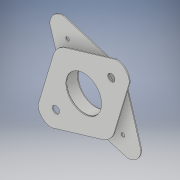
# Autodesk Inventor part: Dampner
Saved by Autodesk Inventor 2019 (Build 230136000, 136)
## iProperties
Created: 2021-06-25
Part Number: Dampner
Material: Generic
Document SubType Name: Modeling
Designer: 91742
Density: 1 g/cm^3
Appearance: Default
Author: 91742
Autodesk Inventor part; units mm, degrees
ref_plane "YZ Plane" through (0, 0, 0) normal (1, 0, 0) x (0, 1, 0)
ref_plane "XZ Plane" through (0, 0, 0) normal (0, 1, 0) x (-1, 0, 0)
ref_plane "XY Plane" through (0, 0, 0) normal (0, 0, 1) x (1, 0, 0)
sketch "Sketch1" plane through (0, 0, 0) normal (0, 0, 1) x (1, 0, 0)
  line L0 (-15.5, 15.261) -> (15.5, -15.739) construction
  line L1 (15.5, 15.261) -> (-15.5, -15.739) construction
  circle A0 centre (15.5, 15.261) radius 2
  circle A1 centre (-15.5, -15.739) radius 2
  line L2 (-25.5, 25.261) -> (25.5, -25.739) construction
  line L3 (25.5, 25.261) -> (-25.5, -25.739) construction
  arc A2 (-25.5, -18.239) -> (-18, -25.739) centre (-18, -18.239) ccw
  arc A3 (25.5, 17.761) -> (18, 25.261) centre (18, 17.761) ccw
  line L4 (-25.5, -18.239) -> (-17.0452, 10.0844)
  line L5 (-10.3234, 16.8062) -> (18, 25.261)
  line L6 (25.5, 17.761) -> (17.0452, -10.5624)
  line L7 (10.3234, -17.2843) -> (-18, -25.739)
  arc A4 (-10.3234, 16.8062) -> (-17.0452, 10.0844) centre (-7.4631, 7.224) ccw
  arc A5 (10.3234, -17.2843) -> (17.0452, -10.5624) centre (7.4631, -7.7021) ccw
  circle A6 centre (0, -0.239) radius 10
  point P0 (0, 0)
  dimension "d0" = 31
  dimension "d1" = 31
  dimension "d2" = 4
  dimension "d3" = 4
  dimension "d6" = 7.5
  dimension "d7" = 10
  dimension "d8" = 20
  constraints: 16 end point, 8 point on circle, 7 centre point, 4 midpoint, 4 point on line, 4 tangent, 3 coincident, 2 equal radius
  measures "d0" distance of L0.end L1.end
  measures "d1" distance of L1.start L0.end
  measures "d2" diameter of A0
  measures "d3" diameter of A1
  measures "d6" radius of A2
  measures "d7" radius of A4
  measures "d8" diameter of A6
extrude "Extrusion1" add sketch "Sketch1" along normal blind 0.5
sketch "Sketch2" plane through (0, 0, 0) normal (0, 0, -1) x (-1, 0, 0)
  circle A0 centre (0, 0) radius 12.5
  circle A1 centre (0, 0) radius 12.5
  circle A2 centre (0, 0) radius 10
  dimension "d11" = 25
  dimension "d12" = 25
  dimension "d13" = 20
  constraints: 3 centre point, 3 coincident
  measures "d11" diameter of A0
  measures "d12" diameter of A1
  measures "d13" diameter of A2
extrude "Extrusion2" add sketch "Sketch2" along normal blind 6
sketch "Sketch3" plane through (0, 0, -6) normal (0, 0, -1) x (-1, 0, 0)
  line L0 (-15.5, 15.261) -> (15.5, -15.739) construction
  line L1 (15.5, 15.261) -> (-15.5, -15.739) construction
  circle A0 centre (15.5, 15.261) radius 1
  circle A1 centre (-15.5, -15.739) radius 1
  line L2 (-25.5, 25.261) -> (25.5, -25.739) construction
  line L3 (25.5, 25.261) -> (-25.5, -25.739) construction
  arc A2 (-25.5, -18.239) -> (-18, -25.739) centre (-18, -18.239) ccw
  arc A3 (25.5, 17.761) -> (18, 25.261) centre (18, 17.761) ccw
  line L4 (-25.5, -18.239) -> (-17.0452, 10.0844)
  line L5 (-10.3234, 16.8062) -> (18, 25.261)
  line L6 (25.5, 17.761) -> (17.0452, -10.5624)
  line L7 (10.3234, -17.2843) -> (-18, -25.739)
  arc A4 (-10.3234, 16.8062) -> (-17.0452, 10.0844) centre (-7.4631, 7.224) ccw
  arc A5 (10.3234, -17.2843) -> (17.0452, -10.5624) centre (7.4631, -7.7021) ccw
  circle A6 centre (0, -0.239) radius 10
  point P0 (0, 0)
  point P1 (0, 0)
  dimension "d16" = 31
  dimension "d17" = 31
  dimension "d18" = 2
  dimension "d19" = 2
  dimension "d20" = 7.5
  dimension "d21" = 10
  dimension "d22" = 20
  constraints: 16 end point, 8 point on circle, 7 centre point, 4 midpoint, 4 point on line, 4 tangent, 3 coincident, 2 equal radius
  measures "d16" distance of L0.end L1.end
  measures "d17" distance of L1.start L0.end
  measures "d18" diameter of A0
  measures "d19" diameter of A1
  measures "d20" radius of A2
  measures "d21" radius of A4
  measures "d22" diameter of A6
extrude "Extrusion3" add sketch "Sketch3" along normal blind 0.5
body "Solid1"
